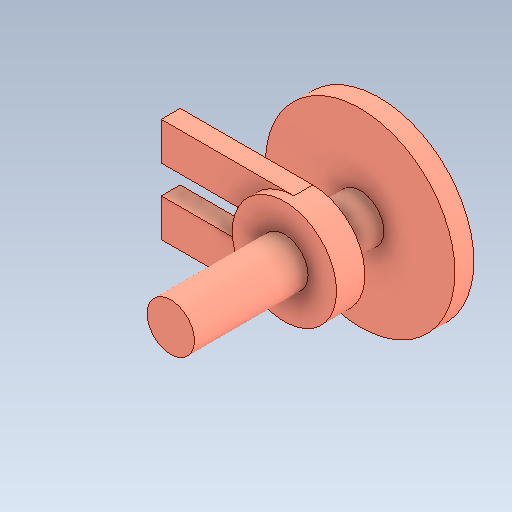
# Autodesk Inventor part: innerGear
Saved by Autodesk Inventor 2020.1 (Build 241239000, 239)
## iProperties
Created: 2020-01-18
Part Number: innerGear
Material: Generic
Document SubType Name: Modeling
Designer: Ali
Density: 1 g/cm^3
Appearance: Default
Author: Ali
Autodesk Inventor part; units mm, degrees
ref_plane "YZ Plane" through (0, 0, 0) normal (1, 0, 0) x (0, 1, 0)
ref_plane "XZ Plane" through (0, 0, 0) normal (0, 1, 0) x (-1, 0, 0)
ref_plane "XY Plane" through (0, 0, 0) normal (0, 0, 1) x (1, 0, 0)
sketch "Sketch1" plane through (0, 0, 0) normal (0, 0, 1) x (1, 0, 0)
  circle A0 centre (0, 0) radius 5
  dimension "d0" = 10
  constraints: 1 centre point, 1 coincident
  measures "d0" diameter of A0
extrude "Extrusion1" add sketch "Sketch1" along normal blind 1
sketch "Sketch2" plane through (0, 0, 1) normal (0, 0, 1) x (1, 0, 0)
  circle A0 centre (0, 0) radius 1.25
  dimension "d3" = 2.5
  constraints: 1 centre point, 1 coincident
  measures "d3" diameter of A0
extrude "Extrusion2" add sketch "Sketch2" along normal blind 10
ref_plane "Work Plane1" through (0, 0, 5) normal (0, 0, 1) x (1, 0, 0)
sketch "Sketch4" plane through (0, 0, 5) normal (0, 0, 1) x (1, 0, 0)
  circle A0 centre (0, 0) radius 1.25 projected
  circle A1 centre (0, 0) radius 2.75
  dimension "d14" = 1.5
  constraints: 1 centre point
  measures "d14" radial gap between concentric circles of A0 A1
extrude "Extrusion4" add sketch "Sketch4" against normal blind 0.5
sketch "Sketch5" plane through (0, 0, 4.5) normal (0, 0, -1) x (-1, 0, 0)
  circle A0 centre (0, 0) radius 2.75 projected
  line L0 (0, 2.75) -> (0, -2.75) construction
  line L1 (0, -2.75) -> (7, -2.75)
  line L2 (7, -2.75) -> (7, 2.75)
  line L3 (7, 2.75) -> (0, 2.75)
  line L4 (0, 2.75) -> (0, -2.75)
  dimension "d18" = 7
  constraints: 10 end point, 2 parallel, 2 point on circle, 1 horizontal, 1 perpendicular, 1 vertical
  measures "d18" distance of L0.end L1.end
extrude "Extrusion5" add sketch "Sketch5" along normal blind 1
sketch "Sketch6" plane through (0, 0, 3.5) normal (0, 0, -1) x (-1, 0, 0)
  line L0 (7, -2.75) -> (7, 2.75) projected
  line L1 (7, 2.75) -> (0, 2.75) projected
  arc A0 (0, 2.75) -> (0, -2.75) centre (0, 0) ccw projected
  line L2 (0, -2.75) -> (7, -2.75) projected
  circle A1 centre (0, 0) radius 1.25 projected
  line L3 (7, 0) -> (5.7457, 0) construction
  line L4 (7, -2.75) -> (7, 2.75) projected
  line L5 (7, -0.75) -> (3, -0.75)
  line L6 (3, -0.75) -> (3, 0.75)
  line L7 (3, 0.75) -> (7, 0.75)
  line L8 (7, 0.75) -> (7, -0.75)
  point P0 (7, 0.75)
  dimension "d21" = 1.5
  dimension "d22" = 0.75
  dimension "d23" = 4
  constraints: 10 end point, 2 horizontal, 2 parallel, 1 midpoint, 1 perpendicular, 1 point on line
  measures "d21" distance of L5.end L6.end
  measures "d22" distance between parallel lines of L3 L7
  measures "d23" distance of L6.end L7.end
extrude "Extrusion6" cut sketch "Sketch6" against normal up to surface (1 mm away) contours L5 L6 L7 L0
equation "\"d1\" = IG_gearThickness"
equation "\"d3\" = IG_shaftDiameter"
equation "\"d4\" = IG_shaftLength"
equation "\"d14\" = IG_skirtOffset"
equation "\"d15\" = IG_skirtThickness"
equation "\"d18\" = IG_extentionLength"
equation "\"d19\" = IG_extentionThickness"
equation "\"d21\" = IG_slitWidth"
equation "\"d22\" = 0.5 * d21"
equation "\"d23\" = IG_slitlength"
equation "\"Wheel_Related_W_\" = 0"
equation "\"W_innerDiameter\" = 35"
equation "\"W_innerDepth\" = 4.5"
equation "\"W_wallThickness\" = 1"
equation "\"W_holesClearance\" = 0.3"
equation "\"W_outerGearHoleDiameter\" = 2.1"
equation "\"W_innerGearHoleDiameter\" = 5.1"
equation "\"TempSpotReserved7\" = 0"
equation "\"TempSpotReserved8\" = 0"
equation "\"TempSpotReserved9\" = 0"
equation "\"TempSpotReserved10\" = 0"
equation "\"TempSpotReserved11\" = 0"
equation "\"TempSpotReserved12\" = 0"
equation "\"TempSpotReserved13\" = 0"
equation "\"TempSpotReserved14\" = 0"
equation "\"TempSpotReserved15\" = 0"
equation "\"TempSpotReserved16\" = 0"
equation "\"TempSpotReserved17\" = 0"
equation "\"TempSpotReserved18\" = 0"
equation "\"TempSpotReserved19\" = 0"
equation "\"TempSpotReserved20\" = 0"
equation "\"Inner_Gear_Related_IG_\" = 0"
equation "\"IG_shaftDiameter\" = 2.5"
equation "\"IG_shaftLength\" = 10"
equation "\"IG_gearThickness\" = 1"
equation "\"TempSpotReserved25\" = 0"
equation "\"TempSpotReserved26\" = 0"
equation "\"TempSpotReserved27\" = 0"
equation "\"TempSpotReserved28\" = 0"
equation "\"TempSpotReserved29\" = 0"
equation "\"TempSpotReserved30\" = 0"
equation "\"TempSpotReserved31\" = 0"
equation "\"TempSpotReserved32\" = 0"
equation "\"TempSpotReserved33\" = 0"
equation "\"TempSpotReserved34\" = 0"
equation "\"TempSpotReserved35\" = 0"
equation "\"TempSpotReserved36\" = 0"
equation "\"TempSpotReserved37\" = 0"
equation "\"TempSpotReserved38\" = 0"
equation "\"TempSpotReserved39\" = 0"
equation "\"TempSpotReserved40\" = 0"
equation "\"Outer_Gear_Related_OG_\" = 0"
equation "\"OG_shaftDiameter\" = 1.5"
equation "\"OG_shaftLength\" = 5"
equation "\"OG_gearThickness\" = 1"
equation "\"TempSpotReserved47\" = 0"
equation "\"TempSpotReserved48\" = 0"
equation "\"TempSpotReserved49\" = 0"
equation "\"TempSpotReserved50\" = 0"
equation "\"TempSpotReserved51\" = 0"
equation "\"TempSpotReserved52\" = 0"
equation "\"TempSpotReserved53\" = 0"
equation "\"TempSpotReserved54\" = 0"
equation "\"TempSpotReserved55\" = 0"
equation "\"TempSpotReserved56\" = 0"
equation "\"TempSpotReserved57\" = 0"
equation "\"TempSpotReserved58\" = 0"
equation "\"TempSpotReserved59\" = 0"
equation "\"TempSpotReserved60\" = 0"
equation "\"Leg_Extensions_Related_LE_\" = 0"
equation "\"LE_baseDiameter\" = 2"
equation "\"LE_maxLength\" = 10.64459"
equation "\"LE_thickness\" = 2"
equation "\"B_bearingThickness\" = 1"
equation "\"TempSpotReserved43\" = 0"
equation "\"TempSpotReserved45\" = 0"
equation "\"Thisisatest\" = 25.4"
equation "\"TempSpotReserved46\" = 0"
equation "\"TempSpotReserved44\" = 0"
equation "\"LE_offsetAboveOuterGear\" = 0"
equation "\"Bearing_Related_B_\" = 0"
equation "\"TempSpotReserved42\" = 0"
equation "\"OG_skirtOffset\" = 1"
equation "\"OG_skirtThickness\" = 1"
equation "\"IG_skirtThickness\" = 0.5"
equation "\"IG_skirtOffset\" = 1.5"
equation "\"d13\" = OG_shaftLength - W_wallThickness"
equation "\"IG_extentionLength\" = 7"
equation "\"IG_extentionThickness\" = 1"
equation "\"IG_slitWidth\" = 1.5"
equation "\"IG_slitlength\" = 4"
body "Solid1"
